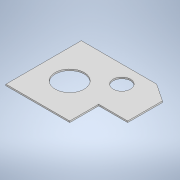
# Autodesk Inventor part: SpacerPlate_Cheese
Saved by Autodesk Inventor 2022.2 (Build 262287030, 287C)
## iProperties
Created: 2023-02-06
Part Number: SpacerPlate_Cheese
Material: Generic
Document SubType Name: Modeling
Designer: jak27277
Density: 1 g/cm^3
Appearance: Default
Author: jak27277
Autodesk Inventor part; units mm, degrees
ref_plane "YZ Plane" through (0, 0, 0) normal (1, 0, 0) x (0, 1, 0)
ref_plane "XZ Plane" through (0, 0, 0) normal (0, 1, 0) x (-1, 0, 0)
ref_plane "XY Plane" through (0, 0, 0) normal (0, 0, 1) x (1, 0, 0)
sketch "Sketch1" plane through (0, 0, 0) normal (0, 1, 0) x (-1, 0, 0)
  circle A0 centre (0, 0) radius 31.75
  line L0 (-139.7, -63.5) -> (-139.7, 12.7)
  line L1 (-139.7, 12.7) -> (-76.2, 12.7)
  line L2 (-76.2, 12.7) -> (-76.2, 76.2)
  line L3 (-76.2, 76.2) -> (63.5, 76.2)
  line L4 (63.5, 76.2) -> (63.5, -88.9)
  line L5 (63.5, -88.9) -> (-101.6, -88.9)
  line L6 (-101.6, -88.9) -> (-139.7, -63.5)
  circle A1 centre (-63.5, -50.8) radius 19.05
  dimension "d0" = 127
  dimension "d1" = 165.1
  dimension "d2" = 63.5
  dimension "d3" = 76.2
  dimension "d4" = 63.5
  dimension "d5" = 63.5
  dimension "d6" = 139.7
  dimension "d7" = 38.1
  dimension "d8" = 165.1
  dimension "d9" = 203.2
  dimension "d10" = 63.5
  dimension "d11" = 38.1
  constraints: 14 end point, 5 perpendicular, 2 centre point, 1 coincident, 1 vertical
  measures "d0" distance from line of A1.centre L4
  measures "d1" distance of L4.end L5.end
  measures "d2" distance from line of point (0, 0) L4
  measures "d3" distance from line of L3 point (0, 0)
  measures "d4" distance of L0.end L1.end
  measures "d5" distance of L1.end L2.end
  measures "d6" distance from line of L0.start L3
  measures "d7" distance from line of L5 A1.centre
  measures "d8" distance of L3.end L4.end
  measures "d9" distance between parallel lines of L0 L4
  measures "d10" diameter of A0
  measures "d11" diameter of A1
extrude "Extrusion1" add sketch "Sketch1" along normal blind 3.175
body "Solid1"
